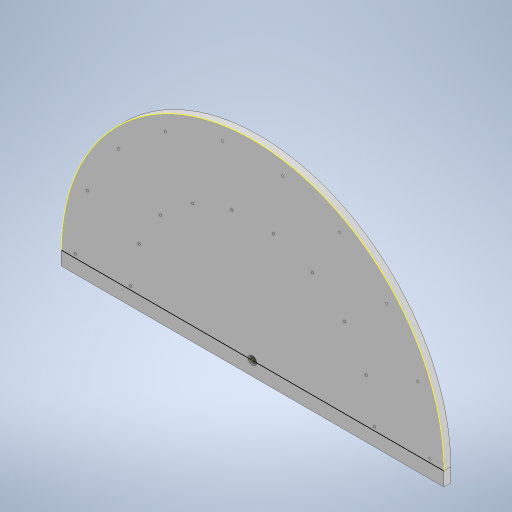
# Autodesk Inventor part: plaque dessus
Saved by Autodesk Inventor 2023 (Build 270158000, 158)
## iProperties
Created: 2022-11-02
Part Number: plaque dessus
Material: Générique
Document SubType Name: Modeling
Designer: Julia
Density: 1 g/cm^3
Appearance: Par défaut
Author: Julia
Autodesk Inventor part; units mm, degrees
ref_plane "YZ Plane" through (0, 0, 0) normal (1, 0, 0) x (0, 1, 0)
ref_plane "XZ Plane" through (0, 0, 0) normal (0, 1, 0) x (-1, 0, 0)
ref_plane "XY Plane" through (0, 0, 0) normal (0, 0, 1) x (1, 0, 0)
sketch "Esquisse1" plane through (0, 0, 0) normal (0, 0, 1) x (1, 0, 0)
  circle A0 centre (0, 0) radius 155
  circle A1 centre (0, 0) radius 275
  line L0 (-275, 0) -> (275, 0)
  line L1 (-155, 0) -> (155, 0)
  circle A2 centre (-175, 5) radius 1.5
  circle A3 centre (175, 5) radius 1.5
  point P0 (-86.6478, -260.9927)
  point P1 (93.3373, -258.6758)
  dimension "d0" = 310
  dimension "d1" = 550
  dimension "d2" = 180
  dimension "d5" = 179.9851
  dimension "d6" = 5
  dimension "d7" = -175
  dimension "d8" = 3
  dimension "d19" = 5
  dimension "d20" = 175
  dimension "d21" = 3
  constraints: 6 point on circle, 4 centre point, 4 end point, 2 coincident, 2 midpoint, 2 point on line, 1 horizontal
  measures "d0" diameter of A0
  measures "d1" diameter of A1
  measures "d2" distance of A1.start A1.end
  measures "d5" horizontal distance of A1.start A1.end
  measures "d6" distance from line of L0 A2.centre
  measures "d7" horizontal distance of point (0, 0) A2.centre
  measures "d8" diameter of A2
  measures "d19" distance from line of L0 A3.centre
  measures "d20" horizontal distance of point (0, 0) A3.centre
  measures "d21" diameter of A3
extrude "Extrusion1" add sketch "Esquisse1" along normal mid plane 10 contours L0 A0 | A0 L0 A1 | A2 | A3 picked at (36.5339, 36.5339) picked at (197.6975, 36.6731)
sketch "Esquisse2" plane through (0, 0, 5) normal (0, 0, 1) x (-1, 0, 0)
  arc A0 (-275, 0) -> (275, 0) centre (0, 0) ccw projected
  line L0 (-275, 0) -> (275, 0)
  constraints: 2 end point, 2 point on circle, 1 horizontal
sketch "Esquisse3" plane through (0, 0, -5) normal (0, 0, -1) x (-1, 0, 0)
  circle A0 centre (175, 5) radius 1.5
  line L0 (275, 0) -> (-275, 0) projected
  point P0 (0, 0)
  point P1 (155, 0)
  dimension "d9" = 175
  dimension "d10" = 5
  dimension "d11" = 3
  constraints: 1 centre point
  measures "d9" horizontal distance of point (0, 0) A0.centre
  measures "d10" distance from line of L0 A0.centre
  measures "d11" diameter of A0
extrude "Extrusion2" cut sketch "Esquisse3" against normal blind 10
sketch "Esquisse4" plane through (0, 0, -5) normal (0, 0, -1) x (-1, 0, 0)
  circle A0 centre (255, 5) radius 1.5
  line L0 (-275, 0) -> (275, 0) projected
  point P0 (0, 0)
  point P1 (155, 0)
  dimension "d14" = 5
  dimension "d15" = 255
  dimension "d16" = 3
  constraints: 1 centre point
  measures "d14" distance from line of L0 A0.centre
  measures "d15" horizontal distance of point (0, 0) A0.centre
  measures "d16" diameter of A0
extrude "Extrusion3" cut sketch "Esquisse4" against normal blind 10
sketch "Esquisse5" plane through (0, 0, 5) normal (0, 0, 1) x (1, 0, 0)
  circle A0 centre (175, 5) radius 1.5
  line L0 (-275, 0) -> (275, 0) projected
  circle A1 centre (255, 5) radius 1.5
  point P0 (0, 0)
  point P1 (0, 0)
  point P2 (0, 0)
  dimension "d22" = 5
  dimension "d23" = 3
  dimension "d24" = 175
  dimension "d25" = 255
  dimension "d26" = 3
  constraints: 2 centre point, 2 midpoint
  measures "d22" distance from line of L0 A0.centre
  measures "d23" diameter of A0
  measures "d24" horizontal distance of point (0, 0) A0.centre
  measures "d25" horizontal distance of point (0, 0) A1.centre
  measures "d26" diameter of A1
extrude "Extrusion4" cut sketch "Esquisse5" against normal blind 10 contours A0
sketch "Esquisse6" plane through (0, 0, 5) normal (0, 0, 1) x (1, 0, 0)
  circle A0 centre (255, 5) radius 1.5
  line L0 (-275, 0) -> (275, 0) projected
  point P0 (0, 0)
  point P1 (0, 0)
  dimension "d31" = 5
  dimension "d32" = 255
  dimension "d33" = 3
  constraints: 1 centre point, 1 midpoint
  measures "d31" distance from line of L0 A0.centre
  measures "d32" horizontal distance of point (0, 0) A0.centre
  measures "d33" diameter of A0
extrude "Extrusion6" cut sketch "Esquisse6" against normal blind 10
sketch "Esquisse7" plane through (0, 0, 5) normal (0, 0, 1) x (1, 0, 0)
  circle A0 centre (163.155, 63.48) radius 1.5
  line L0 (-275, 0) -> (275, 0) projected
  circle A1 centre (237.69, 92.48) radius 1.5
  point P0 (0, 0)
  point P1 (0, 0)
  point P2 (0, 0)
  dimension "d37" = 3
  dimension "d38" = 63.48
  dimension "d39" = 163.155
  dimension "d40" = 92.48
  dimension "d41" = 237.69
  dimension "d42" = 3
  constraints: 2 centre point, 2 midpoint
  measures "d37" diameter of A0
  measures "d38" distance from line of L0 A0.centre
  measures "d39" horizontal distance of point (0, 0) A0.centre
  measures "d40" distance from line of L0 A1.centre
  measures "d41" horizontal distance of point (0, 0) A1.centre
  measures "d42" diameter of A1
extrude "Extrusion7" cut sketch "Esquisse7" against normal blind 10
sketch "Esquisse8" plane through (0, 0, 5) normal (0, 0, 1) x (1, 0, 0)
  circle A0 centre (132.327, 114.625) radius 1.5
  line L0 (-275, 0) -> (275, 0) projected
  circle A1 centre (192.779, 166.991) radius 1.5
  circle A2 centre (86.1, 152.433) radius 1.5
  circle A3 centre (125.43, 222.071) radius 1.5
  circle A4 centre (29.85, 172.5) radius 1.5
  circle A5 centre (43.499, 251.312) radius 1.5
  line L1 (0, 0) -> (0, 275.6506)
  dimension "d45" = 114.625
  dimension "d46" = 132.327
  dimension "d47" = 3
  dimension "d48" = 166.991
  dimension "d49" = 192.779
  dimension "d50" = 3
  dimension "d51" = 152.433
  dimension "d52" = 86.1
  dimension "d53" = 3
  dimension "d54" = 222.071
  dimension "d55" = 125.43
  dimension "d56" = 3
  dimension "d57" = 172.5
  dimension "d58" = 29.85
  dimension "d59" = 3
  dimension "d60" = 251.312
  dimension "d61" = 43.499
  dimension "d62" = 3
  constraints: 6 centre point, 2 end point, 1 vertical, 7 other
  measures "d46" horizontal distance of point (0, 0) A0.centre
  measures "d47" diameter of A0
  measures "d49" horizontal distance of point (0, 0) A1.centre
  measures "d50" diameter of A1
  measures "d52" horizontal distance of point (0, 0) A2.centre
  measures "d53" diameter of A2
  measures "d55" horizontal distance of point (0, 0) A3.centre
  measures "d56" diameter of A3
  measures "d58" horizontal distance of point (0, 0) A4.centre
  measures "d59" diameter of A4
  measures "d61" horizontal distance of L1.start A5.centre
  measures "d62" diameter of A5
extrude "Extrusion8" cut sketch "Esquisse8" against normal blind 10
sketch "Esquisse9" plane through (0, 0, 5) normal (0, 0, 1) x (1, 0, 0)
  circle A0 centre (-163.155, 63.48) radius 1.5
  circle A1 centre (-237.69, 92.48) radius 1.5
  circle A2 centre (-132.327, 114.625) radius 1.5
  circle A3 centre (-192.779, 166.991) radius 1.5
  circle A4 centre (-86.1, 152.433) radius 1.5
  circle A5 centre (-125.43, 222.071) radius 1.5
  circle A6 centre (-29.85, 172.5) radius 1.5
  circle A7 centre (-43.499, 251.312) radius 1.5
  line L0 (-275, 0) -> (275, 0) projected
  point P0 (0, 0)
  point P1 (0, 0)
  point P2 (0, 0)
  point P3 (0, 0)
  point P4 (0, 0)
  point P5 (0, 0)
  point P6 (0, 0)
  point P7 (0, 0)
  point P8 (0, 0)
  dimension "d65" = 63.48
  dimension "d66" = 163.155
  dimension "d67" = 3
  dimension "d68" = 92.48
  dimension "d69" = 237.69
  dimension "d70" = 3
  dimension "d71" = 132.327
  dimension "d72" = 114.625
  dimension "d73" = 3
  dimension "d74" = 166.991
  dimension "d75" = 192.779
  dimension "d76" = 3
  dimension "d77" = 152.433
  dimension "d78" = 86.1
  dimension "d79" = 3
  dimension "d80" = 125.43
  dimension "d81" = 222.071
  dimension "d82" = 3
  dimension "d83" = 29.85
  dimension "d84" = 172.5
  dimension "d85" = 3
  dimension "d86" = 43.499
  dimension "d87" = 251.312
  dimension "d88" = 3
  constraints: 8 centre point, 9 other
  measures "d66" horizontal distance of point (0, 0) A0.centre
  measures "d67" diameter of A0
  measures "d69" horizontal distance of point (0, 0) A1.centre
  measures "d70" diameter of A1
  measures "d71" horizontal distance of point (0, 0) A2.centre
  measures "d73" diameter of A2
  measures "d75" horizontal distance of point (0, 0) A3.centre
  measures "d76" diameter of A3
  measures "d78" horizontal distance of point (0, 0) A4.centre
  measures "d79" diameter of A4
  measures "d80" horizontal distance of point (0, 0) A5.centre
  measures "d82" diameter of A5
  measures "d83" horizontal distance of point (0, 0) A6.centre
  measures "d85" diameter of A6
  measures "d86" horizontal distance of point (0, 0) A7.centre
  measures "d88" diameter of A7
extrude "Extrusion9" cut sketch "Esquisse9" against normal blind 10
sketch "Esquisse11" plane through (0, 0, 5) normal (0, 0, 1) x (1, 0, 0)
  line L0 (275, 0) -> (-275, 0) projected
  line L1 (-275, 0) -> (275, 0)
  line L2 (275, 0) -> (275, -20)
  line L3 (275, -20) -> (-275, -20)
  line L4 (-275, -20) -> (-275, 0)
  point P0 (0, 0)
  dimension "d91" = 20
  constraints: 8 end point, 3 equal length, 1 perpendicular
  measures "d91" distance of L0.start L2.end
extrude "Extrusion10" add sketch "Esquisse11" against normal blind 10
sketch "Esquisse12" plane through (0, 0, 5) normal (0, 0, 1) x (1, 0, 0)
  circle A0 centre (0, 0) radius 6
  dimension "d94" = 12
  constraints: 1 centre point, 1 coincident
  measures "d94" diameter of A0
extrude "Extrusion11" cut sketch "Esquisse12" against normal blind 10
